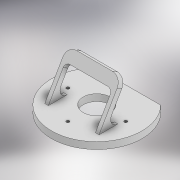
# Autodesk Inventor part: 2
Saved by Autodesk Inventor 2020 (Build 240168000, 168)
## iProperties
Created: 2021-03-27
Part Number: 2
Material: 常规
Document SubType Name: Modeling
Designer: Luorily
Density: 1 g/cm^3
Appearance: 默认
Author: Luorily
Autodesk Inventor part; units mm, degrees
ref_plane "YZ Plane" through (0, 0, 0) normal (1, 0, 0) x (0, 1, 0)
ref_plane "XZ Plane" through (0, 0, 0) normal (0, 1, 0) x (-1, 0, 0)
ref_plane "XY Plane" through (0, 0, 0) normal (0, 0, 1) x (1, 0, 0)
sketch "草图1" plane through (0, 0, 0) normal (0, 1, 0) x (-1, 0, 0)
  circle A0 centre (0, 0) radius 100
  circle A1 centre (0, 0) radius 64 construction
  point P0 (64, 0)
  point P1 (0, 64)
  point P2 (-64, 0)
  dimension "d0" = 200
  dimension "d1" = 128
  constraints: 3 point on circle, 2 centre point, 2 coincident
  measures "d0" diameter of A0
  measures "d1" diameter of A1
extrude "拉伸1" add sketch "草图1" against normal blind 15
hole "孔1" at (-64, 0, 0) at (0, 0, 64) at (64, 0, 0) direction (0, -1, 0) diameter 6.647 end through all thread size "M8x1.25" designation "M8" class "6H" standard "GB Metric profile"
hole "孔2" at (0, 0, 0) direction (0, -1, 0) diameter 60 end through all
sketch "草图2" plane through (0, 0, 0) normal (1, 0, 0) x (0, 1, 0)
  line L0 (0, 55) -> (86.6025, 5)
  line L1 (86.6025, 5) -> (80.6025, -5.3923)
  line L2 (80.6025, -5.3923) -> (24, 27.2872)
  line L3 (0, 27.5) -> (0, 0)
  line L4 (0, 0) -> (0, 13.4308)
  arc A0 (24, 27.2872) -> (0, 13.4308) centre (16, 13.4308) ccw
  line L5 (0, -100) -> (0, 100) projected
  line L6 (0, 55) -> (0, 13.4308)
  point P0 (0, 13.4308)
  dimension "d19" = 55
  dimension "d20" = 100
  dimension "d22" = 12
  dimension "d23" = 0
  dimension "d24" = 16
  constraints: 12 end point, 3 point on circle, 2 perpendicular, 2 tangent, 1 centre point
  measures "d19" distance of point (0, 0) L0.start
  measures "d20" distance of L0.start L0.end
  measures "d22" distance of L0.end L1.end
  measures "d23" distance of point (0, 0) L3.end
  measures "d24" radius of A0
extrude "拉伸2" add sketch "草图2" along normal mid plane 120
sketch "草图3" plane through (-60, 86.6025, 5) normal (0, 0.5, 0.8660254) x (1, 0, 0)
  line L0 (120, -100) -> (0, -100) projected
  line L1 (48.0104, -100) -> (71.9896, -100) projected
  line L2 (120, -100) -> (0, -100) projected
  line L3 (120, -100) -> (112, -100)
  line L4 (112, -100) -> (112, -35)
  line L5 (0, -100) -> (0, -79.2154) projected
  line L6 (0, -100) -> (8, -100)
  line L7 (8, -100) -> (8, -35)
  line L8 (18, -25) -> (102, -25)
  line L9 (112, -100) -> (8, -100)
  arc A0 (18, -25) -> (8, -35) centre (18, -35) ccw
  arc A1 (112, -35) -> (102, -25) centre (102, -35) ccw
  point P0 (60, -72.5)
  point P1 (112, -25)
  point P2 (8, -25)
  dimension "d27" = 8
  dimension "d28" = 75
  dimension "d29" = 8
  dimension "d30" = 75
  dimension "d31" = 10
  constraints: 12 end point, 6 point on line, 4 point on circle, 4 tangent, 3 perpendicular, 2 centre point, 1 collinear, 1 equal radius
  measures "d27" distance of L0.start L3.end
  measures "d28" distance of L3.end point (112, -25)
  measures "d29" distance of L0.end L6.end
  measures "d30" distance of L6.end point (8, -25)
  measures "d31" radius of A0
extrude "拉伸3" cut sketch "草图3" against normal up to surface surface through (0, 0, 0) normal (0, 1, 0)
fillet "圆角1" radius 20 2 edges at (60, 83.6025, -0.1962) (-60, 83.6025, -0.1962)
sketch "草图4" plane through (0, 0, 0) normal (0, 1, 0) x (1, 0, 0)
  circle A0 centre (0, 0) radius 100 projected
  line L0 (0, 0) -> (0, 70)
  line L1 (0, 70) -> (-92.5065, 70)
  line L2 (-92.5065, 70) -> (-88.0231, 170.2178)
  line L3 (-88.0231, 170.2178) -> (67.3235, 163.2683)
  line L4 (67.3235, 163.2683) -> (102.3961, 70)
  line L5 (0, 70) -> (102.3961, 70)
  point P0 (71.4143, 70)
  point P1 (-71.4143, 70)
  dimension "d35" = 70
  constraints: 12 end point, 2 perpendicular, 1 horizontal, 1 vertical
  measures "d35" distance of L0.start L0.end
extrude "拉伸4" cut sketch "草图4" against normal through all contours L5 L1 A0 picked at (-44.3165, 72.9417)
